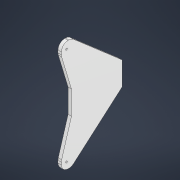
# Autodesk Inventor part: TailHorn
Saved by Autodesk Inventor 2022 (Build 260153000, 153)
## iProperties
Created: 2022-06-02
Part Number: TailHorn
Material: ABS プラスチック
Document SubType Name: Modeling
Designer: hide
Density: 1.06 g/cm^3
Appearance: 滑らか - 白
Mass: 0.3665 g
Surface Area: 7.79377 cm^2
Volume: 0.345754 cm^3
Author: hide
Autodesk Inventor part; units mm, degrees
ref_plane "YZ Plane" through (0, 0, 0) normal (1, 0, 0) x (0, 1, 0)
ref_plane "XZ Plane" through (0, 0, 0) normal (0, 1, 0) x (-1, 0, 0)
ref_plane "XY Plane" through (0, 0, 0) normal (0, 0, 1) x (1, 0, 0)
sketch "スケッチ1" plane through (0, 0, 0) normal (0, 1, 0) x (-1, 0, 0)
  line L0 (-0.5, 7.5) -> (0.5, 7.5)
  line L1 (0.5, 7.5) -> (0.5, -7.5)
  line L2 (0.5, -7.5) -> (-0.5, -7.5)
  line L3 (-0.5, -7.5) -> (-0.5, 7.5)
  line L4 (-0.5, 7.5) -> (0.5, -7.5) construction
  line L5 (0.5, 7.5) -> (-0.5, -7.5) construction
  point P0 (0, 0)
  dimension "d0" = 1
  dimension "d1" = 15
  constraints: 12 end point, 2 midpoint, 2 parallel, 1 horizontal, 1 perpendicular
  measures "d0" distance of L1.end L2.end
  measures "d1" distance of L0.end L1.end
extrude "押し出し1" add sketch "スケッチ1" along normal blind 3.5
sketch "スケッチ2" plane through (0.5, 0, 7.5) normal (1, 0, 0) x (0, 0, -1)
  line L0 (15, 3.5) -> (0, 3.5) projected
  line L1 (-3, 16.5) -> (0, 16.5)
  line L2 (0, 16.5) -> (15, 3.5)
  circle A0 centre (-1.5, 14.5) radius 0.25
  line L3 (-3, 16.5) -> (-3, 13.5)
  line L4 (-3, 13.5) -> (0, 3.5)
  point P0 (7.5, 0)
  point P1 (-1.5, 16.5)
  dimension "d5" = 3
  dimension "d6" = 0.5
  dimension "d7" = 2
  dimension "d11" = 13
  dimension "d12" = 3
  dimension "d13" = 3
  constraints: 8 end point, 1 centre point, 1 horizontal, 1 midpoint, 1 vertical, 1 vertical alignment
  measures "d5" distance of L1.start L1.end
  measures "d6" diameter of A0
  measures "d7" distance from line of L1 A0.centre
  measures "d11" distance between parallel lines of L0 L1
  measures "d12" distance of L1.start L3.end
  measures "d13" horizontal distance of L0.end L3.end
extrude "押し出し2" add sketch "スケッチ2" against normal blind 1
fillet "フィレット1" radius 2 3 edges at (0, 16.5, 10.5) (0, 16.5, 7.5) (0, 13.5, 10.5)
mirror "ミラー1" about plane through (0, 0, 0) normal (0, -1, 0) of "押し出し2", "押し出し1", "フィレット1"
